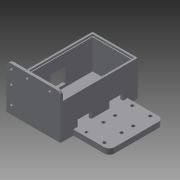
# Autodesk Inventor part: Transmitter Case
Saved by Autodesk Inventor 2014 SP1 (Build 180222100, 222)
## iProperties
Created: 2014-05-13
Part Number: Transmitter Case
Material: Generic
Document SubType Name: Modeling
Designer: Alex
Density: 1 g/cm^3
Appearance: Default
Author: Alex
Autodesk Inventor part; units mm, degrees
ref_plane "YZ Plane" through (0, 0, 0) normal (1, 0, 0) x (0, 1, 0)
ref_plane "XZ Plane" through (0, 0, 0) normal (0, 1, 0) x (-1, 0, 0)
ref_plane "XY Plane" through (0, 0, 0) normal (0, 0, 1) x (1, 0, 0)
sketch "Sketch1" plane through (0, 0, 0) normal (0, 0, 1) x (1, 0, 0)
  line L0 (0, 0) -> (40, 0)
  line L1 (40, 0) -> (40, 60)
  line L2 (40, 60) -> (0, 60)
  line L3 (0, 60) -> (0, 0)
  line L4 (0, 60) -> (0, 70)
  line L5 (0, 0) -> (0, -10)
  line L6 (0, -10) -> (-50, -10)
  line L7 (-50, -10) -> (-50, 70)
  line L8 (-50, 70) -> (0, 70)
  line L9 (0, 70) -> (0, -10)
  line L10 (-50, 70) -> (0, 70)
  line L11 (0, 70) -> (0, 80)
  line L12 (0, 80) -> (-50, 80)
  line L13 (-50, 80) -> (-50, 70)
  line L14 (0, -10) -> (-50, -10)
  line L15 (-50, -10) -> (-50, -20)
  line L16 (-50, -20) -> (0, -20)
  line L17 (0, -20) -> (0, -10)
  line L18 (-50, 70) -> (-25, 70)
  line L19 (-25, 70) -> (-25, 80)
  line L20 (-25, 80) -> (-50, 80)
  line L21 (-50, 80) -> (-50, 70)
  line L22 (-25, 80) -> (0, 80)
  line L23 (0, 80) -> (0, 70)
  line L24 (0, 70) -> (-25, 70)
  line L25 (-25, 70) -> (-25, 80)
  line L26 (-25, 80) -> (-37.5, 80)
  line L27 (-37.5, 80) -> (-37.5, 70)
  line L28 (-37.5, 70) -> (-25, 70)
  line L29 (-25, 70) -> (-25, 80)
  line L30 (-25, 70) -> (-12.5, 70)
  line L31 (-12.5, 70) -> (-12.5, 80)
  line L32 (-12.5, 80) -> (-25, 80)
  line L33 (-25, 80) -> (-25, 70)
  line L34 (-50, 70) -> (-37.5, 70)
  line L35 (-37.5, 70) -> (-37.5, 80)
  line L36 (-37.5, 80) -> (-50, 80)
  line L37 (-50, 80) -> (-50, 70)
  circle A0 centre (-43.75, 75) radius 1.5
  line L38 (-12.5, 70) -> (0, 70)
  line L39 (0, 70) -> (0, 80)
  line L40 (0, 80) -> (-12.5, 80)
  line L41 (-12.5, 80) -> (-12.5, 70)
  circle A1 centre (-6.25, 75) radius 1.5
  line L42 (-50, -10) -> (-25, -10)
  line L43 (-25, -10) -> (-25, -20)
  line L44 (-25, -20) -> (-50, -20)
  line L45 (-50, -20) -> (-50, -10)
  line L46 (-50, -20) -> (-37.5, -20)
  line L47 (-37.5, -20) -> (-37.5, -10)
  line L48 (-37.5, -10) -> (-50, -10)
  line L49 (-50, -10) -> (-50, -20)
  circle A2 centre (-43.75, -15) radius 1.5
  line L50 (-25, -20) -> (0, -20)
  line L51 (0, -20) -> (0, -10)
  line L52 (0, -10) -> (-25, -10)
  line L53 (-25, -10) -> (-25, -20)
  line L54 (0, -10) -> (-12.5, -10)
  line L55 (-12.5, -10) -> (-12.5, -20)
  line L56 (-12.5, -20) -> (0, -20)
  line L57 (0, -20) -> (0, -10)
  circle A3 centre (-6.25, -15) radius 1.5
  dimension "d0" = 40
  dimension "d1" = 60
  dimension "d2" = 10
  dimension "d3" = 10
  dimension "d4" = 50
  dimension "d5" = 10
  dimension "d6" = 10
  dimension "d7" = 3
  dimension "d8" = 3
  dimension "d9" = 3
  dimension "d10" = 3
  constraints: 116 end point, 28 parallel, 14 horizontal, 14 perpendicular, 6 midpoint, 4 centre point, 2 collinear
  measures "d0" distance of L2.end L1.end
  measures "d1" distance of L1.end L0.end
  measures "d2" distance of L2.end L4.end
  measures "d3" distance of L0.start L5.end
  measures "d4" distance of L7.end L8.end
  measures "d5" distance of L11.end L10.end
  measures "d6" distance of L15.end L14.end
  measures "d7" diameter of A0
  measures "d8" diameter of A1
  measures "d9" diameter of A2
  measures "d10" diameter of A3
extrude "Extrusion1" add sketch "Sketch1" along normal blind 4
fillet "Fillet1" radius 8.75 1 edges at (0, -20, 2)
fillet "Fillet2" radius 8.75 1 edges at (-50, -20, 2)
fillet "Fillet3" radius 8.75 1 edges at (0, 80, 2)
fillet "Fillet4" radius 8.75 1 edges at (-50, 80, 2)
sketch "Sketch2" plane through (0, 0, 4) normal (0, 0, 1) x (1, 0, 0)
  line L0 (40, 0) -> (40, 60) projected
  line L1 (40, 60) -> (40, 0)
  line L2 (40, 60) -> (0, 60)
  line L3 (0, 60) -> (0, 46)
  line L4 (0, 46) -> (40, 46)
  line L5 (40, 46) -> (40, 60)
  line L6 (40, 0) -> (0, 0)
  line L7 (0, 0) -> (0, 14)
  line L8 (0, 14) -> (40, 14)
  line L9 (40, 14) -> (40, 0)
  line L10 (40, 46) -> (40, 51)
  line L11 (40, 51) -> (0, 51)
  line L12 (0, 51) -> (0, 41)
  line L13 (0, 41) -> (40, 41)
  line L14 (0, 14) -> (40, 14)
  line L15 (40, 14) -> (40, 19)
  line L16 (40, 19) -> (0, 19)
  line L17 (0, 19) -> (0, 14)
  line L18 (40, 14) -> (0, 14)
  line L19 (0, 14) -> (0, 9)
  line L20 (0, 9) -> (40, 9)
  line L21 (40, 9) -> (40, 14)
  line L22 (0, 60) -> (40, 60)
  line L23 (40, 60) -> (40, 51)
  line L24 (40, 51) -> (0, 51)
  line L25 (0, 51) -> (0, 60)
  line L26 (40, 51) -> (20, 51)
  line L27 (20, 51) -> (20, 60)
  line L28 (20, 60) -> (40, 60)
  line L29 (40, 60) -> (40, 51)
  circle A0 centre (30, 55.5) radius 1.5
  line L30 (0, 51) -> (20, 51)
  line L31 (20, 51) -> (20, 60)
  line L32 (20, 60) -> (0, 60)
  line L33 (0, 60) -> (0, 51)
  circle A1 centre (10, 55.5) radius 1.5
  line L34 (40, 41) -> (0, 41)
  line L35 (0, 41) -> (0, 32)
  line L36 (0, 32) -> (40, 32)
  line L37 (40, 32) -> (40, 41)
  line L38 (0, 32) -> (20, 32)
  line L39 (20, 32) -> (20, 41)
  line L40 (20, 41) -> (0, 41)
  line L41 (0, 41) -> (0, 32)
  line L42 (20, 41) -> (40, 41)
  line L43 (40, 41) -> (40, 32)
  line L44 (40, 32) -> (20, 32)
  line L45 (20, 32) -> (20, 41)
  circle A2 centre (30, 36.5) radius 1.5
  circle A3 centre (10, 36.5) radius 1.5
  line L46 (0, 19) -> (40, 19)
  line L47 (40, 19) -> (40, 28)
  line L48 (40, 28) -> (0, 28)
  line L49 (0, 28) -> (0, 19)
  line L50 (40, 9) -> (0, 9)
  line L51 (0, 9) -> (0, 0)
  line L52 (0, 0) -> (40, 0)
  line L53 (40, 0) -> (40, 9)
  circle A4 centre (10, 23.5) radius 1.5
  circle A5 centre (30, 23.5) radius 1.5
  circle A6 centre (10, 4.5) radius 1.5
  circle A7 centre (30, 4.5) radius 1.5
  dimension "d17" = 14
  dimension "d18" = 14
  dimension "d19" = 5
  dimension "d20" = 10
  dimension "d21" = 5
  dimension "d22" = 5
  dimension "d23" = 3
  dimension "d24" = 3
  dimension "d25" = 9
  dimension "d26" = 3
  dimension "d27" = 3
  dimension "d28" = 9
  dimension "d29" = 3
  dimension "d30" = 3
  dimension "d31" = 3
  dimension "d32" = 3
  constraints: 106 end point, 25 equal length, 14 perpendicular, 12 horizontal, 8 centre point, 7 point on line, 2 midpoint
  measures "d17" distance of L3.end L2.end
  measures "d18" distance of L6.end L7.end
  measures "d19" distance of L4.end L10.end
  measures "d20" distance of L11.end L12.end
  measures "d21" distance of L15.end L14.end
  measures "d22" distance of L19.end L18.end
  measures "d23" diameter of A0
  measures "d24" diameter of A1
  measures "d25" distance of L35.end L34.end
  measures "d26" diameter of A2
  measures "d27" diameter of A3
  measures "d28" distance of L47.end L46.end
  measures "d29" diameter of A4
  measures "d30" diameter of A5
  measures "d31" diameter of A6
  measures "d32" diameter of A7
extrude "Extrusion2" cut sketch "Sketch2" against normal blind 3 contours A0 | A1 | A2 | A3 | A4 | A5 | A6 | A7
sketch "Sketch3" plane through (0, 0, 4) normal (0, 0, 1) x (1, 0, 0)
  circle A0 centre (10, 55.5) radius 1.5 projected
  circle A1 centre (10, 4.5) radius 1.5 projected
  circle A2 centre (10, 23.5) radius 1.5 projected
  circle A3 centre (30, 36.5) radius 1.5 projected
  circle A4 centre (10, 36.5) radius 1.5 projected
  circle A5 centre (30, 23.5) radius 1.5 projected
  circle A6 centre (30, 4.5) radius 1.5 projected
  circle A7 centre (30, 55.5) radius 1.5 projected
  line L0 (0, 60) -> (40, 60)
  line L1 (40, 60) -> (40, 0)
  line L2 (40, 0) -> (0, 0)
  line L3 (0, 0) -> (0, 60)
  circle A8 centre (10, 55.5) radius 1.75
  circle A9 centre (30, 55.5) radius 1.75
  circle A10 centre (10, 36.5) radius 1.75
  circle A11 centre (30, 36.5) radius 1.75
  circle A12 centre (10, 23.5) radius 1.75
  circle A13 centre (30, 23.5) radius 1.75
  circle A14 centre (10, 4.5) radius 1.75
  circle A15 centre (30, 4.5) radius 1.75
  dimension "d116" = 3.5
  dimension "d117" = 3.5
  dimension "d118" = 3.5
  dimension "d119" = 3.5
  dimension "d120" = 3.5
  dimension "d121" = 3.5
  dimension "d122" = 3.5
  dimension "d123" = 3.5
  constraints: 8 centre point, 8 coincident, 8 end point, 2 parallel, 1 horizontal, 1 perpendicular
  measures "d116" diameter of A8
  measures "d117" diameter of A9
  measures "d118" diameter of A10
  measures "d119" diameter of A11
  measures "d120" diameter of A12
  measures "d121" diameter of A13
  measures "d122" diameter of A14
  measures "d123" diameter of A15
extrude "Extrusion3" add sketch "Sketch3" along normal blind 2 contours L0 L1 L2 L3 | A8 | A9 | A10 | A11 | A12 | A13 | A14 | A15
sketch "Sketch4" plane through (0, 0, 0) normal (0, 0, -1) x (-1, 0, 0)
  line L0 (0, 60) -> (-40, 60)
  line L1 (-40, 60) -> (-40, 0)
  line L2 (-40, 0) -> (0, 0)
  line L3 (0, 0) -> (0, 60)
  line L4 (-32.7572, 25.1378) -> (-30.0429, 26.7544)
  line L5 (-30.0429, 26.7544) -> (-27.2857, 25.2121)
  line L6 (-27.2857, 25.2121) -> (-27.2428, 22.0531)
  line L7 (-27.2428, 22.0531) -> (-29.9571, 20.4365)
  line L8 (-29.9571, 20.4365) -> (-32.7143, 21.9789)
  line L9 (-32.7143, 21.9789) -> (-32.7572, 25.1378)
  line L10 (-12.7487, 25.1358) -> (-10.0344, 26.7524)
  line L11 (-10.0344, 26.7524) -> (-7.2772, 25.2101)
  line L12 (-7.2772, 25.2101) -> (-7.2343, 22.0511)
  line L13 (-7.2343, 22.0511) -> (-9.9486, 20.4345)
  line L14 (-9.9486, 20.4345) -> (-12.7058, 21.9769)
  line L15 (-12.7058, 21.9769) -> (-12.7487, 25.1358)
  line L16 (-32.754, 6.1052) -> (-30.0397, 7.7218)
  line L17 (-30.0397, 7.7218) -> (-27.2825, 6.1795)
  line L18 (-27.2825, 6.1795) -> (-27.2397, 3.0206)
  line L19 (-27.2397, 3.0206) -> (-29.954, 1.404)
  line L20 (-29.954, 1.404) -> (-32.7111, 2.9463)
  line L21 (-32.7111, 2.9463) -> (-32.754, 6.1052)
  line L22 (-7.2664, 3.0395) -> (-9.9807, 1.4229)
  line L23 (-9.9807, 1.4229) -> (-12.7379, 2.9652)
  line L24 (-7.3093, 6.1984) -> (-7.2664, 3.0395)
  line L25 (-12.7379, 2.9652) -> (-12.7807, 6.1242)
  line L26 (-10.0664, 7.7408) -> (-7.3093, 6.1984)
  line L27 (-12.7807, 6.1242) -> (-10.0664, 7.7408)
  line L28 (-32.6673, 57.0364) -> (-29.9531, 58.6529)
  line L29 (-29.9531, 58.6529) -> (-27.1959, 57.1106)
  line L30 (-27.1959, 57.1106) -> (-27.153, 53.9517)
  line L31 (-27.153, 53.9517) -> (-29.8673, 52.3351)
  line L32 (-29.8673, 52.3351) -> (-32.6245, 53.8774)
  line L33 (-32.6245, 53.8774) -> (-32.6673, 57.0364)
  line L34 (-7.0966, 53.9496) -> (-9.8109, 52.333)
  line L35 (-9.8109, 52.333) -> (-12.5681, 53.8754)
  line L36 (-7.1395, 57.1086) -> (-7.0966, 53.9496)
  line L37 (-12.5681, 53.8754) -> (-12.6109, 57.0343)
  line L38 (-9.8967, 58.6509) -> (-7.1395, 57.1086)
  line L39 (-12.6109, 57.0343) -> (-9.8967, 58.6509)
  line L40 (-27.3772, 37.9879) -> (-27.3343, 34.829)
  line L41 (-30.1343, 39.5303) -> (-27.3772, 37.9879)
  line L42 (-27.3343, 34.829) -> (-30.0486, 33.2124)
  line L43 (-32.8486, 37.9137) -> (-30.1343, 39.5303)
  line L44 (-30.0486, 33.2124) -> (-32.8057, 34.7547)
  line L45 (-32.8057, 34.7547) -> (-32.8486, 37.9137)
  line L46 (-9.9297, 33.3513) -> (-12.687, 34.8938)
  line L47 (-7.258, 38.1272) -> (-7.2152, 34.968)
  line L48 (-12.687, 34.8938) -> (-12.7299, 38.053)
  line L49 (-10.0154, 39.6697) -> (-7.258, 38.1272)
  line L50 (-12.7299, 38.053) -> (-10.0154, 39.6697)
  line L51 (-7.2152, 34.968) -> (-9.9297, 33.3513)
  point P0 (-30, 23.5955)
  point P1 (-9.9915, 23.5935)
  point P2 (-29.9968, 4.5629)
  point P3 (-10.0236, 4.5818)
  point P4 (-29.9102, 55.494)
  point P5 (-9.8538, 55.492)
  point P6 (-30.0915, 36.3713)
  point P7 (-9.9725, 36.5105)
  dimension "d37" = 5.472
  dimension "d38" = 5.472
  dimension "d41" = 5.472
  dimension "d42" = 5.472
  dimension "d43" = 5.472
  dimension "d44" = 5.472
  dimension "d47" = 5.472
  dimension "d50" = 5.472
  constraints: 104 end point, 2 parallel, 1 horizontal, 1 perpendicular, 104 other
  measures "d37" distance between parallel lines of L8 L5
  measures "d38" distance between parallel lines of L14 L11
  measures "d41" distance between parallel lines of L20 L17
  measures "d42" distance between parallel lines of L23 L26
  measures "d43" distance between parallel lines of L32 L29
  measures "d44" distance between parallel lines of L35 L38
  measures "d47" distance between parallel lines of L44 L41
extrude "Extrusion4" cut sketch "Sketch4" against normal blind 2 contours L4 L5 L6 L7 L8 L9 | L10 L11 L12 L13 L14 L15 | L16 L17 L18 L19 L20 L21 | L22 L23 L25 L27 L26 L24 | L28 L29 L30 L31 L32 L33 | L34 L35 L37 L39 L38 L36 | L40 L42 L44 L45 L43 L41 | L46 L48 L50 L49 L47 L51
fillet "Fillet5" radius 5.75 1 edges at (40, 0, 3)
fillet "Fillet6" radius 5.75 1 edges at (40, 60, 3)
sketch "Sketch5" plane through (0, 0, 4) normal (0, 0, 1) x (1, 0, 0)
  line L0 (0, -11.25) -> (0, 0) projected
  line L1 (0, 71.25) -> (-50, 71.25)
  line L2 (-50, 71.25) -> (-50, -11.25)
  line L3 (-50, -11.25) -> (0, -11.25)
  line L4 (0, -11.25) -> (0, 71.25)
  line L5 (-2, -9.25) -> (-48, -9.25)
  line L6 (-48, -9.25) -> (-2, -9.25)
  line L7 (-2, -9.25) -> (-2, 69.25)
  line L8 (-2, 69.25) -> (-48, 69.25)
  line L9 (-48, 69.25) -> (-48, -9.25)
  line L10 (-48, 69.25) -> (-47, 69.25)
  line L11 (-47, 69.25) -> (-47, 68.25)
  line L12 (-47, 68.25) -> (-48, 68.25)
  line L13 (-48, 68.25) -> (-48, 69.25)
  line L14 (-2, -9.25) -> (-3, -9.25)
  line L15 (-3, -9.25) -> (-3, -8.25)
  line L16 (-3, -8.25) -> (-2, -8.25)
  line L17 (-2, -8.25) -> (-2, -9.25)
  line L18 (-3, -8.25) -> (-47, -8.25)
  line L19 (-47, -8.25) -> (-47, 68.25)
  line L20 (-47, 68.25) -> (-3, 68.25)
  line L21 (-3, 68.25) -> (-3, -8.25)
  dimension "d77" = 1
  dimension "d78" = 1
  dimension "d79" = 1
  dimension "d80" = 1
  constraints: 42 end point, 10 parallel, 6 perpendicular, 5 horizontal
  measures "d77" distance of L11.end L12.end
  measures "d78" distance of L10.end L11.end
  measures "d79" distance of L15.end L16.end
  measures "d80" distance of L14.end L15.end
extrude "Extrusion5" add sketch "Sketch5" along normal blind 35
sketch "Sketch6" plane through (0, -11.25, 0) normal (1, 0, 0) x (0, 0, -1)
  line L0 (-6, 11.25) -> (-16, 11.25)
  line L1 (-16, 11.25) -> (-16, 71.25)
  line L2 (-16, 71.25) -> (-6, 71.25)
  line L3 (-6, 71.25) -> (-6, 11.25)
  dimension "d61" = 10
  constraints: 8 end point, 2 parallel, 1 horizontal, 1 perpendicular
  measures "d61" distance of L1.end L2.end
extrude "Extrusion6" cut sketch "Sketch6" against normal blind 4.5
sketch "Sketch7" plane through (0, -11.25, 0) normal (1, 0, 0) x (0, 0, -1)
  line L0 (-16, 11.25) -> (-6, 11.25)
  line L1 (-6, 11.25) -> (-6, 71.25)
  line L2 (-6, 71.25) -> (-16, 71.25)
  line L3 (-16, 71.25) -> (-16, 11.25)
  line L4 (-6, 71.25) -> (-16, 71.25)
  line L5 (-16, 71.25) -> (-16, 41.25)
  line L6 (-16, 41.25) -> (-6, 41.25)
  line L7 (-6, 41.25) -> (-6, 71.25)
  line L8 (-16, 41.25) -> (-6, 41.25)
  line L9 (-6, 41.25) -> (-6, 31.25)
  line L10 (-6, 31.25) -> (-16, 31.25)
  line L11 (-16, 31.25) -> (-16, 41.25)
  line L12 (-6, 41.25) -> (-16, 41.25)
  line L13 (-16, 41.25) -> (-16, 51.25)
  line L14 (-16, 51.25) -> (-6, 51.25)
  line L15 (-6, 51.25) -> (-6, 41.25)
  line L16 (-6, 71.25) -> (-16, 71.25)
  line L17 (-16, 71.25) -> (-16, 65.9586)
  line L18 (-6, 65.9586) -> (-6, 71.25)
  line L19 (-6, 71.25) -> (-16, 71.25)
  line L20 (-16, 71.25) -> (-16, 66.25)
  line L21 (-16, 66.25) -> (-6, 66.25)
  line L22 (-6, 66.25) -> (-6, 71.25)
  line L23 (-6, 11.25) -> (-16, 11.25)
  line L24 (-16, 11.25) -> (-16, 16.25)
  line L25 (-16, 16.25) -> (-6, 16.25)
  line L26 (-6, 16.25) -> (-6, 11.25)
  dimension "d64" = 10
  dimension "d65" = 10
  dimension "d66" = 5.2914
  dimension "d67" = 5
  dimension "d68" = 5
  constraints: 54 end point, 13 parallel, 7 horizontal, 7 perpendicular, 5 point on line, 1 midpoint
  measures "d64" distance of L8.end L9.end
  measures "d65" distance of L12.end L13.end
  measures "d66" distance of L17.end L16.end
  measures "d67" distance of L20.end L19.end
  measures "d68" distance of L23.end L24.end
extrude "Extrusion7" add sketch "Sketch7" against normal blind 2 contours L3 L25 L1 L0 | L3 L6 L1 L10 | L3 L14 L1 L6 | L3 L2 L1 L21
sketch "Sketch9" plane through (-50, -11.25, 0) normal (-1, 0, 0) x (0, 0, 1)
  line L0 (4, 0) -> (39, 0) projected
  line L1 (4, 82.5) -> (8, 82.5)
  line L2 (8, 82.5) -> (8, 0)
  line L3 (8, 0) -> (4, 0)
  line L4 (4, 0) -> (4, 82.5)
  line L5 (4, 82.5) -> (8, 82.5)
  line L6 (8, 82.5) -> (8, 41.25)
  line L7 (8, 41.25) -> (4, 41.25)
  line L8 (4, 41.25) -> (4, 82.5)
  line L9 (8, 41.25) -> (23, 41.25)
  line L10 (23, 41.25) -> (23, 48.75)
  line L11 (23, 48.75) -> (8, 48.75)
  line L12 (8, 48.75) -> (8, 41.25)
  line L13 (8, 41.25) -> (23, 41.25)
  line L14 (23, 41.25) -> (23, 33.75)
  line L15 (23, 33.75) -> (8, 33.75)
  line L16 (8, 33.75) -> (8, 41.25)
  point P0 (0, 11.25)
  dimension "d71" = 4
  dimension "d72" = 15
  dimension "d73" = 7.5
  dimension "d74" = 7.5
  constraints: 32 end point, 8 parallel, 4 horizontal, 4 perpendicular, 1 midpoint, 1 point on line
  measures "d71" distance of L2.end L3.end
  measures "d72" distance of L11.end L10.end
  measures "d73" distance of L10.end L9.end
  measures "d74" distance of L13.end L14.end
extrude "Extrusion8" cut sketch "Sketch9" against normal blind 2 contours L2 L9 L14 L15 | L2 L11 L10 L9
sketch "Sketch10" plane through (0, 0, 4) normal (0, 0, 1) x (1, 0, 0)
  line L0 (-48, -9.25) -> (-2, -9.25) projected
  line L1 (-2, -9.25) -> (-2, 69.25) projected
  line L2 (-2, 69.25) -> (-48, 69.25) projected
  line L3 (-48, 69.25) -> (-48, -9.25) projected
  line L4 (-48, 69.25) -> (-47, 69.25)
  line L5 (-47, 69.25) -> (-47, 68.25)
  line L6 (-47, 68.25) -> (-48, 68.25)
  line L7 (-48, 68.25) -> (-48, 69.25)
  line L8 (-2, -9.25) -> (-3, -9.25)
  line L9 (-3, -9.25) -> (-3, -8.25)
  line L10 (-3, -8.25) -> (-2, -8.25)
  line L11 (-2, -8.25) -> (-2, -9.25)
  line L12 (-3, -8.25) -> (-47, -8.25)
  line L13 (-47, -8.25) -> (-47, 68.25)
  line L14 (-47, 68.25) -> (-3, 68.25)
  line L15 (-3, 68.25) -> (-3, -8.25)
  point P0 (0, 0)
  dimension "d81" = 1
  dimension "d82" = 1
  dimension "d83" = 1
  dimension "d84" = 1
  constraints: 24 end point, 6 parallel, 3 horizontal, 3 perpendicular
  measures "d81" distance of L5.end L6.end
  measures "d82" distance of L4.end L5.end
  measures "d83" distance of L9.end L10.end
  measures "d84" distance of L8.end L9.end
extrude "Extrusion9" add sketch "Sketch10" along normal blind 33 contours L3 L6 L13 L12 L9 L0 | L9 L10 L1 L0 | L3 L2 L5 L6 | L15 L14 L5 L2 L1 L10
sketch "Sketch11" plane through (-2, 5, 6) normal (1, 0, 0) x (0, 0, -1)
  line L0 (-10, 0) -> (0, 0) projected
  line L1 (0, 0) -> (0, 15) projected
  line L2 (-10, 0) -> (0, 0)
  line L3 (0, 0) -> (0, 15)
  line L4 (0, 15) -> (-10, 15)
  line L5 (-10, 15) -> (-10, 0)
  point P0 (6, -5)
  constraints: 8 end point, 2 parallel, 1 horizontal, 1 perpendicular
extrude "Extrusion10" cut sketch "Sketch11" against normal blind 6
sketch "Sketch12" plane through (-2, 40, 16) normal (1, 0, 0) x (0, 0, -1)
  line L0 (10, 15) -> (0, 15) projected
  line L1 (0, 15) -> (0, 0) projected
  line L2 (0, 0) -> (10, 0)
  line L3 (10, 0) -> (10, 15)
  line L4 (10, 15) -> (0, 15)
  line L5 (0, 15) -> (0, 0)
  point P0 (16, -40)
  constraints: 8 end point, 2 parallel, 1 horizontal, 1 perpendicular
extrude "Extrusion11" cut sketch "Sketch12" against normal blind 6
sketch "Sketch13" plane through (-48, 22.5, 23) normal (-1, 0, 0) x (0, 0, 1)
  line L0 (-15, 0) -> (0, 0) projected
  line L1 (0, 0) -> (0, 15) projected
  line L2 (-15, 0) -> (0, 0)
  line L3 (0, 0) -> (0, 15)
  line L4 (0, 15) -> (-15, 15)
  line L5 (-15, 15) -> (-15, 0)
  point P0 (-23, -22.5)
  constraints: 8 end point, 2 parallel, 1 horizontal, 1 perpendicular
extrude "Extrusion12" cut sketch "Sketch13" against normal blind 22.25
delete faces "Delete Face1" heal yes whole lump no faces at (-19.5833, 76.6667, 4) (-30.4167, 80, 2.6667) (-0.3887, 73.8291, 1.3333) (-44.4467, 79.3951, 1.3333)
delete faces "Delete Face2" heal yes whole lump no faces at (-30.4167, -16.6667, 4) (-1.5204, -16.1791, 1.3333) (-30.4167, -20, 1.3333) (-48.8277, -15.625, 1.3333)
sketch "Sketch14" plane through (-50, -11.25, 0) normal (0, -1, 0) x (1, 0, 0)
  line L0 (50, 0) -> (-10, 0)
  line L1 (-10, 0) -> (-10, 49)
  line L2 (-10, 49) -> (50, 49)
  line L3 (50, 49) -> (50, 0)
  dimension "d93" = 60
  dimension "d94" = 49
  constraints: 8 end point, 2 parallel, 1 horizontal, 1 perpendicular
  measures "d93" distance of L1.end L2.end
  measures "d94" distance of L0.end L1.end
extrude "Extrusion13" add sketch "Sketch14" along normal blind 3
sketch "Sketch15" plane through (-50, -11.25, 0) normal (0, 1, 0) x (1, 0, 0)
  circle A0 centre (-5, -44) radius 1.75
  line L0 (50, -49) -> (0, -49)
  line L1 (0, -49) -> (0, -39)
  line L2 (0, -39) -> (50, -39)
  line L3 (50, -39) -> (50, -49)
  line L4 (0, -39) -> (25, -39)
  line L5 (25, -39) -> (25, -49)
  line L6 (25, -49) -> (0, -49)
  line L7 (0, -49) -> (0, -39)
  line L8 (25, -49) -> (50, -49)
  line L9 (50, -49) -> (50, -39)
  line L10 (50, -39) -> (25, -39)
  line L11 (25, -39) -> (25, -49)
  circle A1 centre (37.5, -44) radius 1.75
  circle A2 centre (12.5, -44) radius 1.75
  line L12 (0, -39) -> (-10, -39)
  line L13 (-10, -39) -> (-10, 0)
  line L14 (-10, 0) -> (0, 0)
  line L15 (0, 0) -> (0, -39)
  line L16 (-10, 0) -> (0, 0)
  line L17 (0, 0) -> (0, -19.5)
  line L18 (0, -19.5) -> (-10, -19.5)
  line L19 (-10, -19.5) -> (-10, 0)
  line L20 (0, -19.5) -> (-10, -19.5)
  line L21 (-10, -19.5) -> (-10, -39)
  line L22 (-10, -39) -> (0, -39)
  line L23 (0, -39) -> (0, -19.5)
  circle A3 centre (-5, -29.25) radius 1.75
  circle A4 centre (-5, -9.75) radius 1.75
  point P0 (50, 0)
  dimension "d97" = 3.5
  dimension "d98" = 3.5
  dimension "d99" = 3.5
  dimension "d100" = 3.5
  dimension "d101" = 3.5
  constraints: 48 end point, 12 parallel, 6 horizontal, 6 perpendicular, 5 centre point, 2 midpoint
  measures "d97" diameter of A0
  measures "d98" diameter of A1
  measures "d99" diameter of A2
  measures "d100" diameter of A3
  measures "d101" diameter of A4
extrude "Extrusion14" cut sketch "Sketch15" against normal blind 3.25 contours A0 | A1 | A2 | A3 | A4
fillet "Fillet7" radius 5.25 1 edges at (-60, -12.75, 49)
fillet "Fillet8" radius 5.5 1 edges at (0, -12.75, 49)
sketch "Sketch17" plane through (-50, 71.25, 0) normal (-1, 0, 0) x (0, 0, 1)
  line L0 (23, -48.75) -> (8, -48.75) projected
  line L1 (8, -48.75) -> (8, -33.75) projected
  line L2 (8, -33.75) -> (23, -33.75) projected
  line L3 (23, -33.75) -> (23, -48.75) projected
  line L4 (8, -33.75) -> (7, -33.75)
  line L5 (7, -33.75) -> (7, -32.75)
  line L6 (7, -32.75) -> (8, -32.75)
  line L7 (8, -32.75) -> (8, -33.75)
  line L8 (23, -48.75) -> (24, -48.75)
  line L9 (24, -48.75) -> (24, -49.75)
  line L10 (24, -49.75) -> (23, -49.75)
  line L11 (23, -49.75) -> (23, -48.75)
  line L12 (7, -32.75) -> (24, -32.75)
  line L13 (24, -32.75) -> (24, -49.75)
  line L14 (24, -49.75) -> (7, -49.75)
  line L15 (7, -49.75) -> (7, -32.75)
  point P0 (0, -71.25)
  dimension "d106" = 1
  dimension "d107" = 1
  dimension "d108" = 1
  dimension "d109" = 1
  constraints: 24 end point, 6 parallel, 3 horizontal, 3 perpendicular
  measures "d106" distance of L5.end L6.end
  measures "d107" distance of L4.end L5.end
  measures "d108" distance of L9.end L10.end
  measures "d109" distance of L8.end L9.end
extrude "Extrusion15" cut sketch "Sketch17" against normal blind 4.75 contours L11 L14 L15 L4 L1 L0 | L3 L2 L7 L12 L13 L8 | L8 L9 L10 L11 | L4 L5 L6 L7
sketch "Sketch18" plane through (0, 60, 0) normal (1, 0, 0) x (0, 0, -1)
  line L0 (-6, -55) -> (-16, -55) projected
  line L1 (-16, -5) -> (-6, -5) projected
  line L2 (-16, -20) -> (-13, -20)
  line L3 (-13, -20) -> (-13, -5)
  line L4 (-13, -5) -> (-16, -5)
  line L5 (-16, -5) -> (-16, -20)
  line L6 (-16, -40) -> (-13, -40)
  line L7 (-13, -40) -> (-13, -55)
  line L8 (-13, -55) -> (-16, -55)
  line L9 (-16, -55) -> (-16, -40)
  dimension "d112" = 3
  dimension "d113" = 3
  constraints: 16 end point, 4 parallel, 2 horizontal, 2 perpendicular, 2 point on line
  measures "d112" distance of L4.end L3.end
  measures "d113" distance of L7.end L8.end
extrude "Extrusion16" add sketch "Sketch18" against normal blind 3
sketch "Sketch19" plane through (0, 0, 6) normal (0, 0, 1) x (1, 0, 0)
  circle A0 centre (30, 55.5) radius 1.5 projected
  circle A1 centre (30, 4.5) radius 1.5 projected
  circle A2 centre (30, 23.5) radius 1.5 projected
  circle A3 centre (10, 36.5) radius 1.5 projected
  circle A4 centre (30, 36.5) radius 1.5 projected
  circle A5 centre (10, 23.5) radius 1.5 projected
  circle A6 centre (10, 55.5) radius 1.5 projected
  circle A7 centre (10, 55.5) radius 1.5
  circle A8 centre (10, 4.5) radius 1.5
  circle A9 centre (10, 23.5) radius 1.5
  circle A10 centre (30, 36.5) radius 1.5
  circle A11 centre (10, 36.5) radius 1.5
  circle A12 centre (30, 23.5) radius 1.5
  circle A13 centre (30, 4.5) radius 1.5
  circle A14 centre (30, 55.5) radius 1.5
  circle A15 centre (10, 55.5) radius 1.75
  circle A16 centre (30, 55.5) radius 1.75
  circle A17 centre (10, 36.5) radius 1.75
  circle A18 centre (30, 36.5) radius 1.75
  circle A19 centre (10, 23.5) radius 1.75
  circle A20 centre (30, 23.5) radius 1.75
  circle A21 centre (10, 4.5) radius 1.75
  circle A22 centre (30, 4.5) radius 1.75
  dimension "d124" = 3.5
  dimension "d125" = 3.5
  dimension "d126" = 3.5
  dimension "d127" = 3.5
  dimension "d128" = 3.5
  dimension "d129" = 3.5
  dimension "d130" = 3.5
  dimension "d131" = 3.5
  constraints: 16 centre point, 8 coincident
  measures "d124" diameter of A15
  measures "d125" diameter of A16
  measures "d126" diameter of A17
  measures "d127" diameter of A18
  measures "d128" diameter of A19
  measures "d129" diameter of A20
  measures "d130" diameter of A21
  measures "d131" diameter of A22
extrude "Extrusion17" cut sketch "Sketch19" against normal blind 9.25 contours A15 | A16 | A17 | A18 | A19 | A20 | A22
sketch "Sketch20" plane through (34.25, 60, 0) normal (0, 0, -1) x (-1, 0, 0)
  line L0 (1.4014, -22.0863) -> (4.1157, -20.4697) projected
  line L1 (4.1157, -20.4697) -> (6.8728, -22.0121) projected
  line L2 (6.8728, -22.0121) -> (6.9157, -25.171) projected
  line L3 (6.9157, -25.171) -> (4.2014, -26.7876) projected
  line L4 (4.2014, -26.7876) -> (1.4443, -25.2453) projected
  line L5 (1.4443, -25.2453) -> (1.4014, -22.0863) projected
  line L6 (27.1105, -2.8914) -> (27.1534, -6.0504) projected
  line L7 (27.1534, -6.0504) -> (24.4391, -7.667) projected
  line L8 (24.4391, -7.667) -> (21.6819, -6.1246) projected
  line L9 (21.6819, -6.1246) -> (21.6391, -2.9657) projected
  line L10 (21.6391, -2.9657) -> (24.3533, -1.3491) projected
  line L11 (24.3533, -1.3491) -> (27.1105, -2.8914) projected
  line L12 (26.9836, -56.9605) -> (24.2693, -58.5771) projected
  line L13 (24.2693, -58.5771) -> (21.5121, -57.0348) projected
  line L14 (21.5121, -57.0348) -> (21.4693, -53.8758) projected
  line L15 (21.4693, -53.8758) -> (24.1836, -52.2592) projected
  line L16 (24.1836, -52.2592) -> (26.9407, -53.8016) projected
  line L17 (26.9407, -53.8016) -> (26.9836, -56.9605) projected
  line L18 (1.5357, -38.0211) -> (1.4928, -34.8622) projected
  line L19 (1.4928, -34.8622) -> (4.2071, -33.2456) projected
  line L20 (4.2071, -33.2456) -> (6.9643, -34.7879) projected
  line L21 (6.9643, -34.7879) -> (7.0072, -37.9469) projected
  line L22 (7.0072, -37.9469) -> (4.2929, -39.5635) projected
  line L23 (4.2929, -39.5635) -> (1.5357, -38.0211) projected
  line L24 (26.9728, -34.7899) -> (27.0157, -37.9489) projected
  line L25 (27.0157, -37.9489) -> (24.3014, -39.5655) projected
  line L26 (24.3014, -39.5655) -> (21.5442, -38.0231) projected
  line L27 (21.5442, -38.0231) -> (21.5013, -34.8642) projected
  line L28 (21.5013, -34.8642) -> (24.2156, -33.2476) projected
  line L29 (24.2156, -33.2476) -> (26.9728, -34.7899) projected
  line L30 (1.496, -53.8948) -> (4.2103, -52.2782) projected
  line L31 (4.2103, -52.2782) -> (6.9675, -53.8205) projected
  line L32 (6.9675, -53.8205) -> (7.0103, -56.9794) projected
  line L33 (7.0103, -56.9794) -> (4.296, -58.596) projected
  line L34 (4.296, -58.596) -> (1.5389, -57.0537) projected
  line L35 (1.5389, -57.0537) -> (1.496, -53.8948) projected
  line L36 (1.5827, -2.9636) -> (4.2969, -1.3471) projected
  line L37 (4.2969, -1.3471) -> (7.0541, -2.8894) projected
  line L38 (7.0541, -2.8894) -> (7.097, -6.0483) projected
  line L39 (7.097, -6.0483) -> (4.3827, -7.6649) projected
  line L40 (4.3827, -7.6649) -> (1.6255, -6.1226) projected
  line L41 (1.6255, -6.1226) -> (1.5827, -2.9636) projected
  line L42 (21.5201, -21.947) -> (24.2346, -20.3303) projected
  line L43 (24.2346, -20.3303) -> (26.992, -21.8728) projected
  line L44 (26.992, -21.8728) -> (27.0348, -25.032) projected
  line L45 (27.0348, -25.032) -> (24.3203, -26.6487) projected
  line L46 (24.3203, -26.6487) -> (21.563, -25.1062) projected
  line L47 (21.563, -25.1062) -> (21.5201, -21.947) projected
  line L48 (4.3827, -0.7856) -> (7.6368, -2.6644)
  line L49 (7.6368, -2.6644) -> (7.6368, -6.4219)
  line L50 (7.6368, -6.4219) -> (4.3827, -8.3007)
  line L51 (4.3827, -8.3007) -> (1.1286, -6.4219)
  line L52 (1.1286, -6.4219) -> (1.1286, -2.6644)
  line L53 (1.1286, -2.6644) -> (4.3827, -0.7856)
  line L54 (24.3533, -0.7856) -> (27.5432, -2.6272)
  line L55 (27.5432, -2.6272) -> (27.5432, -6.3105)
  line L56 (27.5432, -6.3105) -> (24.3533, -8.1522)
  line L57 (24.3533, -8.1522) -> (21.1635, -6.3105)
  line L58 (21.1635, -6.3105) -> (21.1635, -2.6272)
  line L59 (21.1635, -2.6272) -> (24.3533, -0.7856)
  line L60 (4.2969, -19.9913) -> (7.3586, -21.759)
  line L61 (7.3586, -21.759) -> (7.3586, -25.2943)
  line L62 (7.3586, -25.2943) -> (4.2969, -27.0619)
  line L63 (4.2969, -27.0619) -> (1.2353, -25.2943)
  line L64 (1.2353, -25.2943) -> (1.2353, -21.759)
  line L65 (1.2353, -21.759) -> (4.2969, -19.9913)
  line L66 (24.2346, -19.7622) -> (27.4947, -21.6444)
  line L67 (27.4947, -21.6444) -> (27.4947, -25.4089)
  line L68 (27.4947, -25.4089) -> (24.2346, -27.2911)
  line L69 (24.2346, -27.2911) -> (20.9745, -25.4089)
  line L70 (20.9745, -25.4089) -> (20.9745, -21.6444)
  line L71 (20.9745, -21.6444) -> (24.2346, -19.7622)
  line L72 (4.2103, -32.8244) -> (7.3447, -34.634)
  line L73 (7.3447, -34.634) -> (7.3447, -38.2533)
  line L74 (7.3447, -38.2533) -> (4.2103, -40.0629)
  line L75 (4.2103, -40.0629) -> (1.0759, -38.2533)
  line L76 (1.0759, -38.2533) -> (1.0759, -34.634)
  line L77 (1.0759, -34.634) -> (4.2103, -32.8244)
  line L78 (24.2346, -32.8244) -> (27.369, -34.634)
  line L79 (27.369, -34.634) -> (27.369, -38.2533)
  line L80 (27.369, -38.2533) -> (24.2346, -40.0629)
  line L81 (24.2346, -40.0629) -> (21.1002, -38.2533)
  line L82 (21.1002, -38.2533) -> (21.1002, -34.634)
  line L83 (21.1002, -34.634) -> (24.2346, -32.8244)
  line L84 (4.2969, -51.9132) -> (7.3808, -53.6937)
  line L85 (7.3808, -53.6937) -> (7.3808, -57.2547)
  line L86 (7.3808, -57.2547) -> (4.2969, -59.0352)
  line L87 (4.2969, -59.0352) -> (1.213, -57.2547)
  line L88 (1.213, -57.2547) -> (1.213, -53.6937)
  line L89 (1.213, -53.6937) -> (4.2969, -51.9132)
  line L90 (24.2156, -51.613) -> (27.5435, -53.5714)
  line L91 (27.5435, -53.5714) -> (27.5114, -57.4326)
  line L92 (27.5114, -57.4326) -> (24.1515, -59.3354)
  line L93 (24.1515, -59.3354) -> (20.8236, -57.3771)
  line L94 (20.8236, -57.3771) -> (20.8557, -53.5158)
  line L95 (20.8557, -53.5158) -> (24.2156, -51.613)
  point P0 (4.3827, -4.5431)
  point P1 (24.3533, -4.4689)
  point P2 (4.2969, -23.5266)
  point P3 (24.2346, -23.5266)
  point P4 (4.2103, -36.4437)
  point P5 (24.2346, -36.4437)
  point P6 (4.2969, -55.4742)
  point P7 (24.1836, -55.4742)
  constraints: 96 end point, 104 other
extrude "Extrusion18" cut sketch "Sketch20" against normal blind 2.5
body "Solid1"
